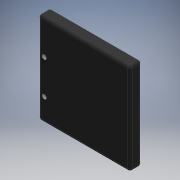
# Autodesk Inventor part: 升降板
Saved by Autodesk Inventor 2017 (Build 210142000, 142)
## iProperties
Part Number: 升降板
Material: 常规
Document SubType Name: Modeling
Designer: PANDA
Density: 1 g/cm^3
Appearance: 默认
Mass: 9.73602 g
Surface Area: 31.2078 cm^2
Volume: 9.73602 cm^3
Author: PANDA
Autodesk Inventor part; units mm, degrees
ref_plane "YZ Plane" through (0, 0, 0) normal (1, 0, 0) x (0, 1, 0)
ref_plane "XZ Plane" through (0, 0, 0) normal (0, 1, 0) x (-1, 0, 0)
ref_plane "XY Plane" through (0, 0, 0) normal (0, 0, 1) x (1, 0, 0)
sketch "草图1" plane through (0, 0, 0) normal (0, 1, 0) x (-1, 0, 0)
  line L0 (40, 40) -> (-40, 40)
  line L1 (-40, 40) -> (-40, -40)
  line L2 (-40, -40) -> (40, -40)
  line L3 (40, -40) -> (40, 40)
  point P0 (0, 0)
  dimension "d13" = 80
  dimension "d14" = 80
  constraints: 8 end point, 2 parallel, 1 horizontal, 1 perpendicular
  measures "d13" distance of L2.end L1.end
  measures "d14" distance of L1.end L0.end
extrude "拉伸1" add sketch "草图1" along normal blind 10
fillet "圆角1" radius 2 12 edges at (-40, 5, -40) (-40, 5, 40) (-40, 0, 0) (-40, 10, 0) (40, 5, -40) (0, 0, -40) (0, 10, -40) (40, 5, 40) (40, 0, 0) (40, 10, 0) (0, 0, 40) (0, 10, 40)
sketch "草图4" plane through (0, 0, 0) normal (0, -1, 0) x (1, 0, 0)
  circle A0 centre (-35, -20) radius 2
  point P0 (0, 0)
  dimension "d15" = 4
  constraints: 1 centre point
  measures "d15" diameter of A0
extrude "拉伸4" cut sketch "草图4" against normal through all
sketch "草图5" plane through (0, 0, 0) normal (0, -1, 0) x (1, 0, 0)
  circle A0 centre (-35, 10) radius 2
  point P0 (0, 0)
  dimension "d18" = 4
  constraints: 1 centre point
  measures "d18" diameter of A0
extrude "拉伸5" cut sketch "草图5" against normal through all
